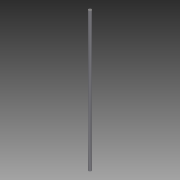
# Autodesk Inventor part: YShaft
Saved by Autodesk Inventor 2016 (Build 200138000, 138)
## iProperties
Category: Hardware
Created: 2014-08-15
Part Number: YShaft
Material: Steel, Alloy
Document SubType Name: Modeling
Designer: t_clevj
Density: 7.73 g/cm^3
Appearance: Semi-Polished
Mass: 143.764 g
Surface Area: 93.9965 cm^2
Volume: 18.5982 cm^3
Catalog Web Link: http://us.misumi-ec.com/vona2/detail/110300000120/
Vendor: Misumi
Stock Number: PSFJ8-366
Author: Jack
Title: Y Axis Shaft
Comments: 366mm Long
Autodesk Inventor part; units mm, degrees
ref_plane "YZ Plane" through (0, 0, 0) normal (1, 0, 0) x (0, 1, 0)
ref_plane "XZ Plane" through (0, 0, 0) normal (0, 1, 0) x (-1, 0, 0)
ref_plane "XY Plane" through (0, 0, 0) normal (0, 0, 1) x (1, 0, 0)
sketch "Sketch1" plane through (0, 0, 0) normal (0, 0, 1) x (1, 0, 0)
  circle A0 centre (0, 0) radius 4
  dimension "d0" = 8
  constraints: 1 centre point, 1 coincident
  measures "d0" diameter of A0
extrude "Extrusion1" add sketch "Sketch1" along normal blind 370
body "Solid1"
